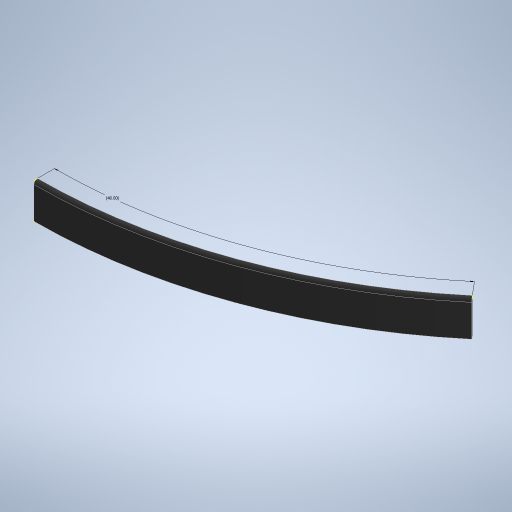
# Autodesk Inventor part: side band
Saved by Autodesk Inventor 2024 (Build 280153000, 153)
## iProperties
Created: 2025-11-15
Part Number: side band
Material: Rubber
Document SubType Name: Modeling
Designer: garys
Density: 0.93 g/cm^3
Appearance: Rubber - Black
Author: garys
Autodesk Inventor part; units mm, degrees
ref_plane "YZ Plane" through (0, 0, 0) normal (1, 0, 0) x (0, 1, 0)
ref_plane "XZ Plane" through (0, 0, 0) normal (0, 1, 0) x (-1, 0, 0)
ref_plane "XY Plane" through (0, 0, 0) normal (0, 0, 1) x (1, 0, 0)
sketch "Sketch1" plane through (0, 0, 0) normal (1, 0, 0) x (0, 1, 0)
  line L0 (0, 0) -> (12.7, 0)
  line L1 (12.7, 0) -> (12.7, -1.27)
  line L2 (12.7, -1.27) -> (0, -1.27)
  line L3 (0, -1.27) -> (0, 0)
  line L4 (0, -1.27) -> (0, -179.07)
  line L5 (0, -179.07) -> (48.3251, -179.07)
  dimension "d0" = 12.7
  dimension "d1" = 1.27
  dimension "d3" = 177.8
  constraints: 12 end point, 2 horizontal, 2 parallel, 1 perpendicular, 1 vertical
  measures "d0" distance of L1.end L2.end
  measures "d1" distance of L0.end L1.end
  measures "d3" distance of L2.end L4.end
sketch "Sketch2" plane through (0, 0, 0) normal (0, 1, 0) x (-1, 0, 0)
  point P0 (0, 0)
revolve "Revolution1" add sketch "Sketch1" angle 40 about axis through (0, 0, -179.07) along (0, 1, 0)
sketch "Sketch4" plane through (0, 12.7, -179.07) normal (0, 1, 0) x (0.9397, 0, -0.342)
  line L0 (-60.8112, -167.0773) -> (-61.2455, -168.2708) projected
  line L1 (60.8112, -167.0773) -> (61.2455, -168.2708) projected
  dimension "d5" = 40
  measures "d5" angle of L0 L1
fillet "Fillet1" radius 1.27 1 edges at (61.2455, 12.7, -10.7992)
body "Solid1"
